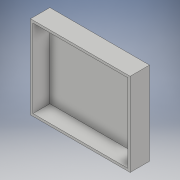
# Autodesk Inventor part: Temporary Platform
Saved by Autodesk Inventor 2018 (Build 220112000, 112)
## iProperties
Created: 2019-01-12
Part Number: Temporary Platform
Material: Generic
Document SubType Name: Modeling
Designer: maste
Density: 1 g/cm^3
Appearance: Default
Author: maste
Autodesk Inventor part; units mm, degrees
ref_plane "YZ Plane" through (0, 0, 0) normal (1, 0, 0) x (0, 1, 0)
ref_plane "XZ Plane" through (0, 0, 0) normal (0, 1, 0) x (-1, 0, 0)
ref_plane "XY Plane" through (0, 0, 0) normal (0, 0, 1) x (1, 0, 0)
sketch "Sketch1" plane through (0, 0, 0) normal (0, 0, 1) x (1, 0, 0)
  line L0 (0, 0) -> (784.098, 0)
  line L1 (784.098, 0) -> (784.098, 655.574)
  line L2 (784.098, 655.574) -> (0, 655.574)
  line L3 (0, 655.574) -> (0, 0)
  dimension "d0" = 784.098
  dimension "d1" = 655.574
  constraints: 8 end point, 2 parallel, 1 horizontal, 1 perpendicular
  measures "d0" distance of L2.end L1.end
  measures "d1" distance of L1.end L0.end
extrude "Extrusion1" add sketch "Sketch1" along normal blind 19.05
sketch "Sketch2" plane through (0, 0, 19.05) normal (0, 0, 1) x (1, 0, 0)
  line L0 (784.098, 0) -> (784.098, 655.574) projected
  line L1 (0, 0) -> (784.098, 0)
  line L2 (784.098, 0) -> (784.098, 655.574)
  line L3 (784.098, 655.574) -> (0, 655.574)
  line L4 (0, 655.574) -> (0, 0)
  line L5 (19.05, 636.524) -> (765.048, 636.524)
  line L6 (765.048, 636.524) -> (765.048, 19.05)
  line L7 (765.048, 19.05) -> (19.05, 19.05)
  line L8 (19.05, 19.05) -> (19.05, 636.524)
  dimension "d4" = 19.05
  constraints: 16 end point, 4 parallel, 2 perpendicular, 1 horizontal, 3 other
  measures "d4" distance between parallel lines of L3 L5
extrude "Extrusion2" add sketch "Sketch2" along normal blind 133.35
body "Solid1"
